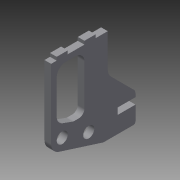
# Autodesk Inventor part: Handle 27021014
Saved by Autodesk Inventor 2015 (Build 190159000, 159)
## iProperties
Created: 2011-12-01
Part Number: Handle 27021014
Document SubType Name: Modeling
Designer: user
Density: 1 g/cm^3
Material: Generic
Appearance: Default
Author: user
Autodesk Inventor part; units mm, degrees
ref_plane "YZ Plane" through (0, 0, 0) normal (1, 0, 0) x (0, 1, 0)
ref_plane "XZ Plane" through (0, 0, 0) normal (0, 1, 0) x (-1, 0, 0)
ref_plane "XY Plane" through (0, 0, 0) normal (0, 0, 1) x (1, 0, 0)
sketch "Sketch1" plane through (0, 0, 0) normal (0, 0, 1) x (1, 0, 0)
  line L0 (51, -62.5841) -> (51, 0)
  line L1 (21, 0) -> (21, 3)
  line L2 (21, 3) -> (11, 3)
  line L3 (11, 3) -> (11, 0)
  line L4 (36, 0) -> (36, 3)
  line L5 (36, 3) -> (46, 3)
  line L6 (46, 3) -> (46, 0)
  line L7 (51, 0) -> (46, 0)
  line L8 (36, 0) -> (21, 0)
  line L9 (11, 0) -> (0, 0)
  line L10 (-9, -69.8) -> (-25, -69.8)
  line L11 (-9, -64) -> (-25, -64)
  line L12 (-9, -69.8) -> (-9, -64)
  line L13 (-25, -69.8) -> (-25, -82.8)
  line L14 (29, -5) -> (38, -5)
  line L15 (46, -13) -> (46, -43.9388)
  line L16 (21, -50) -> (21, -13)
  arc A0 (29, -5) -> (21, -13) centre (29, -13) ccw
  arc A1 (46, -13) -> (38, -5) centre (38, -13) ccw
  line L17 (4.2384, -84.7068) -> (44.0172, -72.118)
  line L18 (26, -55) -> (30.1184, -55)
  line L19 (31.8285, -54.6985) -> (40.7362, -51.4563)
  arc A2 (21, -50) -> (26, -55) centre (26, -50) ccw
  arc A3 (30.1184, -55) -> (31.8285, -54.6985) centre (30.1184, -50) ccw
  arc A4 (40.7362, -51.4563) -> (46, -43.9388) centre (38, -43.9388) ccw
  arc A5 (44.0172, -72.118) -> (51, -62.5841) centre (41, -62.5841) ccw
  circle A6 centre (17.1651, -70.1271) radius 5
  circle A7 centre (41, -62.5841) radius 5
  line L20 (-25, -64) -> (-25, -61.0711)
  line L21 (-23.5355, -57.5355) -> (-2.9289, -36.9289)
  line L22 (0, -29.8579) -> (0, 0)
  arc A8 (-2.9289, -36.9289) -> (0, -29.8579) centre (-10, -29.8579) ccw
  arc A9 (-23.5355, -57.5355) -> (-25, -61.0711) centre (-20, -61.0711) ccw
  line L23 (-23, -84.8) -> (3.635, -84.8)
  arc A10 (-25, -82.8) -> (-23, -84.8) centre (-23, -82.8) ccw
  arc A11 (3.635, -84.8) -> (4.2384, -84.7068) centre (3.635, -82.8) ccw
  point P0 (0, 0)
  point P1 (16, 3)
  point P2 (41, 3)
  point P3 (51, -69.9082)
  point P4 (-25, -84.8)
  point P5 (46, -49.5404)
  point P6 (21, -55)
  point P7 (31, -55)
  point P8 (-25, -59)
  point P9 (0, -34)
  dimension "d17" = 10
  dimension "d18" = 3
  dimension "d20" = 10
  dimension "d21" = 3
  dimension "d22" = 5
  dimension "d23" = 15
  dimension "d24" = 3
  dimension "d25" = 3
  dimension "d75" = 90
  dimension "d129" = 64
  dimension "d130" = 16
  dimension "d131" = 60
  dimension "d139" = 5.8
  dimension "d148" = 5
  dimension "d149" = 5
  dimension "d152" = 8
  dimension "d162" = 10
  dimension "d164" = 160
  dimension "d167" = 55
  dimension "d169" = 5
  dimension "d170" = 5
  dimension "d171" = 8
  dimension "d173" = 10
  dimension "d184" = 5
  dimension "d185" = 30
  dimension "d186" = 135
  dimension "d187" = 10
  dimension "d188" = 5
  dimension "d189" = 25
  dimension "d190" = 15
  dimension "d191" = 25
  dimension "d192" = 2
  constraints: 48 end point, 20 point on circle, 20 tangent, 14 point on line, 12 centre point, 4 horizontal, 3 horizontal alignment, 3 parallel, 3 perpendicular, 2 equal radius, 2 midpoint, 1 coincident, 1 vertical alignment
  measures "d17" distance of L1.end L2.end
  measures "d18" distance of L2.end L3.end
  measures "d20" distance of L4.end L5.end
  measures "d21" distance of L5.end L6.end
  measures "d22" distance between parallel lines of L0 L6
  measures "d23" distance of L4.start L1.start
  measures "d24" distance of L1.start L1.end
  measures "d25" distance of L4.start L4.end
  measures "d75" angle of L7 L6
  measures "d129" distance between parallel lines of L11 L9
  measures "d130" distance of L11.start L11.end
  measures "d131" distance between parallel lines of L12 L0
  measures "d139" distance of L10.start L11.start
  measures "d148" distance between parallel lines of L0 L15
  measures "d149" distance between parallel lines of L14 L8
  measures "d152" radius of A0
  measures "d162" distance of point (21, -55) point (31, -55)
  measures "d164" angle of L18 L19
  measures "d167" distance between parallel lines of L18 L9
  measures "d169" radius of A2
  measures "d170" radius of A3
  measures "d171" radius of A4
  measures "d173" radius of A5
  measures "d184" distance of L11.end point (-25, -59)
  measures "d185" distance from line of point (0, -34) L11
  measures "d186" angle of L20 L21
  measures "d187" radius of A8
  measures "d188" radius of A9
  measures "d189" distance between parallel lines of L15 L16
  measures "d190" distance of L10.end point (-25, -84.8)
  measures "d191" distance of A6.centre A5.centre
  measures "d192" radius of A10
extrude "Extrusion10" add sketch "Sketch1" along normal blind 6
body "Solid10"
